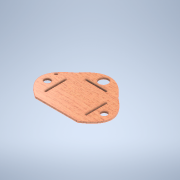
# Autodesk Inventor part: CarTop_V2
Saved by Autodesk Inventor 2022.2 (Build 262287000, 287)
## iProperties
Created: 2022-11-22
Part Number: CarTop_V2
Material: Wood (Oak)
Document SubType Name: Modeling
Designer: jaege
Density: 0.76 g/cm^3
Appearance: Red Oak - Natural Low Gloss
Author: jaege
Autodesk Inventor part; units mm, degrees
ref_plane "YZ Plane" through (0, 0, 0) normal (1, 0, 0) x (0, 1, 0)
ref_plane "XZ Plane" through (0, 0, 0) normal (0, 1, 0) x (-1, 0, 0)
ref_plane "XY Plane" through (0, 0, 0) normal (0, 0, 1) x (1, 0, 0)
sketch "Sketch2" plane through (0, 0, 0) normal (0, 1, 0) x (-1, 0, 0)
  line L0 (-49, 47) -> (49, 47)
  line L1 (49, 47) -> (49, -47)
  line L2 (49, -47) -> (-49, -47)
  line L3 (-49, -47) -> (-49, 47)
  line L4 (-49, 47) -> (49, -47) construction
  line L5 (49, 47) -> (-49, -47) construction
  line L6 (49, -23) -> (45, -23)
  line L7 (45, -23) -> (45, 27)
  line L8 (45, 27) -> (49, 27)
  line L9 (49, 27) -> (49, -23)
  line L10 (-49, -23) -> (-45, -23)
  line L11 (-45, -23) -> (-45, 27)
  line L12 (-45, 27) -> (-49, 27)
  line L13 (-49, 27) -> (-49, -23)
  line L14 (25, -47) -> (-25, -47)
  line L15 (-25, -47) -> (-25, -43)
  line L16 (-25, -43) -> (25, -43)
  line L17 (25, -43) -> (25, -47)
  line L18 (0, -65.8) -> (0, 65.8)
  line L19 (68.6, 0) -> (-68.6, 0)
  line L20 (49, 2) -> (-45, 2) construction
  point P0 (0, 0)
  point P1 (-25, -47)
  dimension "d7" = 98
  dimension "d8" = 94
  dimension "d5" = 4
  dimension "d6" = 50
  dimension "d3" = 4
  dimension "d4" = 50
  dimension "d1" = 50
  dimension "d2" = 4
  dimension "d0" = 2
  constraints: 42 end point, 8 parallel, 5 perpendicular, 4 horizontal, 4 midpoint, 3 point on line, 1 horizontal alignment, 2 other
  measures "d7" distance of L1.end L2.end
  measures "d8" distance of L0.end L1.end
  measures "d5" distance of L7.end L8.end
  measures "d6" distance of L6.end L7.end
  measures "d3" distance of L12.end L11.end
  measures "d4" distance of L11.end L10.end
  measures "d1" distance of L15.end L16.end
  measures "d2" distance of L14.end L15.end
  measures "d0" distance between parallel lines of L19 L20
extrude "Extrusion1" add sketch "Sketch2" along normal blind 4 contours L0 L18 L19 L11 L12 L3 | L0 L1 L8 L7 L19 L18 | L19 L7 L6 L1 L2 L17 L16 L18 | L18 L16 L15 L2 L3 L10 L11 L19
sketch "Sketch3" plane through (0, 4, 0) normal (0, 1, 0) x (1, 0, 0)
  circle A0 centre (0, 62.5) radius 11
  line L0 (49, 47) -> (25, 47) construction
  line L1 (-25, 47) -> (-49, 47) construction
  spline S0 degree 2 poles (-49, 47) (0, 109) (49, 47) knots 0 0 0 1 1 1
  line L2 (-25, 43) -> (-25, 47) projected
  line L3 (-25, 47) -> (25, 47)
  circle A1 centre (66, -2) radius 7.5
  line L4 (49, 23) -> (49, 47) construction
  line L5 (49, -47) -> (49, -27) construction
  spline S1 degree 2 poles (49, 47) (117.0133, -2.6879) (49, -47) knots 0 0 0 1 1 1
  line L6 (45, 23) -> (49, 23) projected
  line L7 (49, 23) -> (49, -27)
  line L8 (25, 43) -> (-25, 43) projected
  line L9 (0, 43) -> (0, -47)
  line L10 (-49, -47) -> (49, -47) projected
  circle A2 centre (-66, -2) radius 7.5
  spline S2 degree 2 poles (-49, 47) (-117.0133, -2.6879) (-49, -47) knots 0 0 0 1 1 1
  line L11 (-49, 23) -> (-49, -27)
  line L12 (-49, 47) -> (-49, 23) construction
  line L13 (-49, -27) -> (-49, -47) construction
  line L14 (-49, 23) -> (-45, 23) projected
  line L15 (-45, 23) -> (-45, -27) projected
  line L16 (-45, -27) -> (-49, -27) projected
  line L17 (45, -27) -> (45, 23) projected
  line L18 (49, -27) -> (45, -27) projected
  line L19 (25, 47) -> (25, 43) projected
  line L20 (-68.3848, 24.8284) -> (-65.5563, 22)
  line L21 (-65.5563, 22) -> (-69.799, 17.7574)
  line L22 (-69.799, 17.7574) -> (-72.6274, 20.5858)
  line L23 (-72.6274, 20.5858) -> (-68.3848, 24.8284)
  point P0 (0, 0)
  point P1 (0, 78)
  point P2 (83, -2)
  point P3 (-83, -2)
  dimension "d12" = 22
  dimension "d13" = 15.5
  dimension "d14" = 15.5
  dimension "d17" = 17
  dimension "d18" = 15
  dimension "d19" = 17
  dimension "d20" = 2
  dimension "d21" = 6
  dimension "d22" = 4
  dimension "d23" = 25
  dimension "d25" = 135
  dimension "d26" = 11
  constraints: 16 end point, 4 symmetric about line, 3 centre point, 2 midpoint, 2 parallel, 2 perpendicular, 2 vertical alignment, 1 horizontal alignment, 10 other
  measures "d12" diameter of A0
  measures "d13" distance from line of L0 A0.centre
  measures "d14" distance of A0.centre point (0, 78)
  measures "d17" distance from line of L4 A1.centre
  measures "d18" diameter of A1
  measures "d19" distance of point (83, -2) A1.centre
  measures "d20" vertical distance of point (0, 0) A1.centre
  measures "d21" distance of L20.end L21.end
  measures "d22" distance of L20.start L20.end
  measures "d23" vertical distance of L20.end L1.end
  measures "d25" angle of L14 L21
  measures "d26" distance from line of L11.start L21
extrude "Extrusion2" add sketch "Sketch3" against normal blind 4
body "Solid1"
